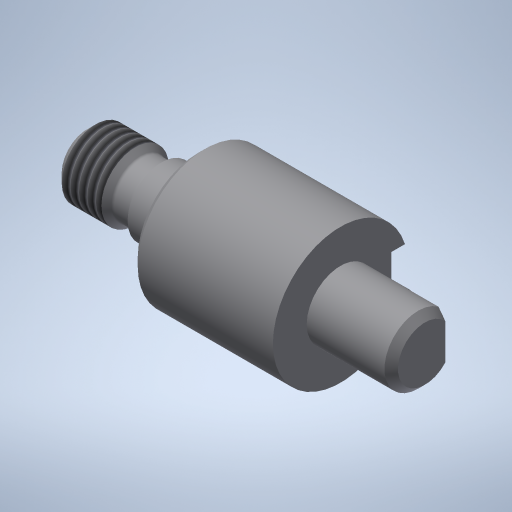
# Autodesk Inventor part: Вал
Saved by Autodesk Inventor 2023.2 (Build 272271030, 271C)
## iProperties
Created: 2017-03-09
Part Number: Вал
Material: Типовые
Document SubType Name: Modeling
Designer: Cтас
Density: 1 g/cm^3
Appearance: По умолчанию
Author: Cтас
Autodesk Inventor part; units mm, degrees
ref_plane "YZ Plane" through (0, 0, 0) normal (1, 0, 0) x (0, 1, 0)
ref_plane "XZ Plane" through (0, 0, 0) normal (0, 1, 0) x (-1, 0, 0)
ref_plane "XY Plane" through (0, 0, 0) normal (0, 0, 1) x (1, 0, 0)
sketch "Эскиз1" plane through (0, 0, 0) normal (0, 0, 1) x (1, 0, 0)
  line L0 (-20, 0) -> (120, 0) projected
  line L1 (0, -4) -> (0, 24) projected
  line L2 (0, 0) -> (0, 10)
  line L3 (0, 10) -> (16, 10)
  line L4 (16, 10) -> (16, 8.25)
  line L5 (16, 8.25) -> (22, 8.25)
  line L6 (22, 8.25) -> (22, 10)
  line L7 (22, 10) -> (33, 10)
  line L8 (33, 10) -> (33, 20)
  line L9 (33, 20) -> (75, 20)
  line L10 (75, 20) -> (75, 10)
  line L11 (75, 10) -> (100, 10)
  line L12 (100, 10) -> (100, 0)
  line L13 (100, 0) -> (0, 0)
  dimension "d0" = 20
  dimension "d1" = 16.5
  dimension "d2" = 20
  dimension "d3" = 6
  dimension "d4" = 22
  dimension "d5" = 100
  dimension "d6" = 25
  dimension "d7" = 42
  dimension "d8" = 40
  dimension "d9" = 20
  constraints: 24 end point, 5 parallel, 3 collinear, 3 perpendicular, 1 midpoint, 1 point on line
  measures "d0" diameter of L3 L13
  measures "d1" diameter of L5 L13
  measures "d2" diameter of L7 L13
  measures "d3" distance of L4.end L5.end
  measures "d4" distance between parallel lines of L1 L6
  measures "d5" distance between parallel lines of L1 L12
  measures "d6" distance between parallel lines of L10 L12
  measures "d7" distance between parallel lines of L8 L10
  measures "d8" diameter of L9 L13
  measures "d9" diameter of L11 L13
revolve "Вращение1" add sketch "Эскиз1" angle 360 about axis through (-10, 0, 0) along (1, 0, 0)
thread "Резьба1" size "M20x2.5" class "6g" standard "ANSI Metric M Profile" full length
chamfer "Фаска1" distance 2.5 angle 45 1 edges at (0, -10, 0)
sketch "Эскиз2" plane through (0, 0, 0) normal (0, 0, 1) x (1, 0, 0)
  line L0 (0, 7.5) -> (2.5, 10) projected
  line L1 (2.5, 10) -> (16, 10) projected
  line L2 (16, 10) -> (16, 8.25) projected
  line L3 (16, 8.25) -> (22, 8.25) projected
  line L4 (22, 8.25) -> (22, 10) projected
  line L5 (22, 10) -> (33, 10) projected
  line L6 (33, 10) -> (33, 20) projected
  line L7 (33, 20) -> (75, 20) projected
  line L8 (75, 20) -> (75, 10) projected
  line L9 (75, 10) -> (100, 10) projected
  line L10 (100, 10) -> (100, -10) projected
  line L11 (100, -10) -> (75, -10) projected
  line L12 (75, -10) -> (75, -20) projected
  line L13 (75, -20) -> (33, -20) projected
  line L14 (33, -20) -> (33, -10) projected
  line L15 (33, -10) -> (22, -10) projected
  line L16 (22, -10) -> (22, -8.25) projected
  line L17 (22, -8.25) -> (16, -8.25) projected
  line L18 (16, -8.25) -> (16, -10) projected
  line L19 (16, -10) -> (2.5, -10) projected
  line L20 (2.5, -10) -> (0, -7.5) projected
  line L21 (0, -7.5) -> (0, 7.5) projected
  line L22 (16, 8.25) -> (14.25, 10)
  line L23 (16, 10) -> (14.25, 10)
  line L24 (16, 10) -> (16, 8.25)
  line L25 (-20, 0) -> (120, 0) projected
  point P0 (0, 0)
  constraints: 6 end point, 1 collinear, 1 parallel
revolve "Вращение2" cut sketch "Эскиз2" angle 360 about axis through (-10, 0, 0) along (1, 0, 0) contours L1 L2 L22
fillet "Сопряжение1" radius 1 1 edges at (16, -8.25, 0)
fillet "Сопряжение2" radius 1.6 1 edges at (22, -8.25, 0)
chamfer "Фаска2" distance 2 angle 45 1 edges at (33, -20, 0)
chamfer "Фаска3" distance 2 angle 45 1 edges at (100, -10, 0)
sketch "Эскиз3" plane through (0, 0, 0) normal (0, 0, 1) x (1, 0, 0)
  line L0 (0, 7.5) -> (2.5, 10) projected
  line L1 (2.5, 10) -> (14.25, 10) projected
  line L2 (14.25, 10) -> (15.7071, 8.5429) projected
  arc A0 (15.7071, 8.5429) -> (16.4142, 8.25) centre (16.4142, 9.25) ccw projected
  line L3 (16.4142, 8.25) -> (20.4, 8.25) projected
  arc A1 (20.4, 8.25) -> (22, 9.85) centre (20.4, 9.85) ccw projected
  line L4 (22, 9.85) -> (22, 10) projected
  line L5 (22, 10) -> (33, 10) projected
  line L6 (33, 10) -> (33, 18) projected
  line L7 (33, 18) -> (35, 20) projected
  line L8 (35, 20) -> (75, 20) projected
  line L9 (75, 20) -> (75, 10) projected
  line L10 (75, 10) -> (98, 10) projected
  line L11 (98, 10) -> (100, 8) projected
  line L12 (100, 8) -> (100, -8) projected
  line L13 (100, -8) -> (98, -10) projected
  line L14 (98, -10) -> (75, -10) projected
  line L15 (75, -10) -> (75, -20) projected
  line L16 (75, -20) -> (35, -20) projected
  line L17 (35, -20) -> (33, -18) projected
  line L18 (33, -18) -> (33, -10) projected
  line L19 (33, -10) -> (22, -10) projected
  line L20 (22, -10) -> (22, -9.85) projected
  arc A2 (22, -9.85) -> (20.4, -8.25) centre (20.4, -9.85) ccw projected
  line L21 (20.4, -8.25) -> (16.4142, -8.25) projected
  arc A3 (16.4142, -8.25) -> (15.7071, -8.5429) centre (16.4142, -9.25) ccw projected
  line L22 (15.7071, -8.5429) -> (14.25, -10) projected
  line L23 (14.25, -10) -> (2.5, -10) projected
  line L24 (2.5, -10) -> (0, -7.5) projected
  line L25 (0, -7.5) -> (0, 7.5) projected
  line L26 (100, 6) -> (88, 6)
  line L27 (88, 6) -> (88, 10)
  line L28 (88, 10) -> (88, 15)
  line L29 (88, 15) -> (103, 15)
  line L30 (103, 15) -> (100, 6)
  point P0 (0, 0)
  dimension "d25" = 12
  dimension "d26" = 16
  dimension "d27" = 5
  dimension "d28" = 15
  constraints: 10 end point, 3 perpendicular, 2 point on line, 1 collinear
  measures "d25" distance between parallel lines of L12 L27
  measures "d26" distance between parallel lines of L14 L26
  measures "d27" distance of L27.end L28.end
  measures "d28" distance of L28.end L29.end
extrude "Выдавливание1" cut sketch "Эскиз3" along normal mid plane 100 contours L28 L29 L30 L12 L11 L10 | L10 L11 L12 L26 L27
sketch "Эскиз4" plane through (75, 0, 0) normal (1, 0, 0) x (0, 0, -1)
  line L0 (-6, 15) -> (6, 15)
  line L1 (0, -28) -> (0, 28) projected
  line L2 (-6, 15) -> (-6, 25)
  line L3 (-6, 25) -> (6, 25)
  line L4 (6, 25) -> (6, 15)
  circle A0 centre (0, 0) radius 10 projected
  circle A1 centre (0, 0) radius 20 projected
  line L5 (0, 20) -> (6, 20) construction
  dimension "d31" = 10
  dimension "d32" = 12
  dimension "d33" = 5
  constraints: 10 end point, 2 parallel, 2 perpendicular, 1 horizontal, 1 midpoint, 1 point on line, 1 symmetric about line, 1 vertical alignment, 1 other
  measures "d31" distance of L0.start L2.end
  measures "d32" distance of L2.end L3.end
  measures "d33" distance between parallel lines of L0 L5
extrude "Выдавливание2" cut sketch "Эскиз4" against normal blind 14 contours L2 A1 L1 L0 | L1 A1 L4 L0 | L2 L3 L1 A1 | L1 L3 L4 A1
sketch "Эскиз5" plane through (75, 15, 6) normal (0, 1, 0) x (1, 0, 0)
  line L0 (-14, 12) -> (-14, 0) projected
  circle A0 centre (-14, 6) radius 6
  point P0 (-75, 6)
  constraints: 1 midpoint, 1 vertical alignment, 2 other
extrude "Выдавливание3" cut sketch "Эскиз5" along normal blind 15
